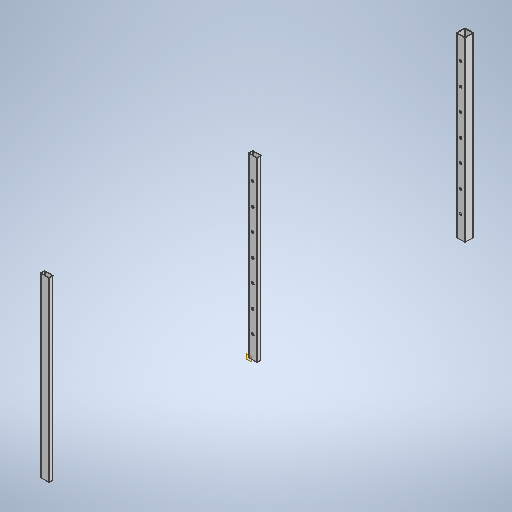
# Autodesk Inventor part: korlat1
Saved by Autodesk Inventor 2025.2 (Build 292293000, 293)
## iProperties
Created: 2025-08-30
Part Number: korlat1
Material: Generic
Document SubType Name: Modeling
Designer: MB
Density: 1 g/cm^3
Appearance: Default
Author: MB
Autodesk Inventor part; units mm, degrees
ref_plane "YZ Plane" through (0, 0, 0) normal (1, 0, 0) x (0, 1, 0)
ref_plane "XZ Plane" through (0, 0, 0) normal (0, 1, 0) x (-1, 0, 0)
ref_plane "XY Plane" through (0, 0, 0) normal (0, 0, 1) x (1, 0, 0)
sketch "Sketch1" plane through (0, 0, 0) normal (0, 1, 0) x (-1, 0, 0)
  line L0 (2, 0) -> (38, 0)
  line L1 (40, 2) -> (40, 38)
  line L2 (38, 40) -> (2, 40)
  line L3 (0, 38) -> (0, 2)
  line L4 (5, 37) -> (35, 37)
  line L5 (37, 35) -> (37, 5)
  line L6 (35, 3) -> (5, 3)
  line L7 (3, 5) -> (3, 35)
  arc A0 (5, 37) -> (3, 35) centre (5, 35) ccw
  arc A1 (37, 35) -> (35, 37) centre (35, 35) ccw
  arc A2 (3, 5) -> (5, 3) centre (5, 5) ccw
  arc A3 (35, 3) -> (37, 5) centre (35, 5) ccw
  arc A4 (38, 0) -> (40, 2) centre (38, 2) ccw
  arc A5 (0, 2) -> (2, 0) centre (2, 2) ccw
  arc A6 (2, 40) -> (0, 38) centre (2, 38) ccw
  arc A7 (40, 38) -> (38, 40) centre (38, 38) ccw
  point P0 (0, 0)
  point P1 (40, 40)
  point P2 (40, 0)
  point P3 (0, 40)
  dimension "d0" = 40
  dimension "d1" = 40
  dimension "d2" = 3
  dimension "d3" = 3
  dimension "d4" = 3
  dimension "d5" = 3
  dimension "d6" = 2
  constraints: 16 end point, 16 point on circle, 16 tangent, 8 centre point, 8 point on line, 7 equal radius, 4 parallel, 2 horizontal, 2 perpendicular
  measures "d0" distance of point (0, 40) point (40, 40)
  measures "d1" distance of point (40, 40) point (40, 0)
  measures "d2" distance between parallel lines of L0 L6
  measures "d3" distance between parallel lines of L3 L7
  measures "d4" distance between parallel lines of L1 L5
  measures "d5" distance between parallel lines of L2 L4
  measures "d6" radius of A0
extrude "Extrusion1" add sketch "Sketch1" along normal blind 800
sketch "Sketch2" plane through (-38, 0, 40) normal (0, 0, 1) x (1, 0, 0)
  line L0 (0, 0) -> (0, 800) projected
  line L1 (-2, 0) -> (-2, 800) projected
  line L2 (0, 800) -> (36, 800) projected
  point P0 (38, 0)
  point P1 (18, 700)
  point P2 (18, 800)
  point P3 (18, 600)
  point P4 (18, 500)
  point P5 (18, 400)
  point P6 (18, 300)
  point P7 (18, 200)
  point P8 (18, 100)
  dimension "d10" = 20
  dimension "d11" = 100
  dimension "d14" = 100
  constraints: 1 midpoint, 1 vertical, 6 other
  measures "d10" distance from line of L1 point (18, 700)
  measures "d11" distance of point (18, 800) point (18, 700)
  measures "d14" distance of point (18, 700) point (18, 600)
hole "Hole1" at (-20, 600, 40) at (-20, 500, 40) at (-20, 400, 40) at (-20, 300, 40) at (-20, 200, 40) at (-20, 100, 40) at (-20, 700, 40) direction (0, 0, -1) diameter 12 depth 8 tip angle 118
sketch "Sketch3" plane through (0, 0, 0) normal (0, 1, 0) x (-1, 0, 0)
  line L0 (2, 960) -> (38, 960)
  line L1 (40, 962) -> (40, 978)
  line L2 (38, 980) -> (2, 980)
  line L3 (0, 978) -> (0, 962)
  line L4 (4, 962) -> (36, 962)
  line L5 (38, 964) -> (38, 976)
  line L6 (36, 978) -> (4, 978)
  line L7 (2, 976) -> (2, 964)
  line L8 (38, 40) -> (2, 40) projected
  line L9 (0, 38) -> (0, 2) projected
  arc A0 (2, 964) -> (4, 962) centre (4, 964) ccw
  arc A1 (0, 962) -> (2, 960) centre (2, 962) ccw
  arc A2 (38, 960) -> (40, 962) centre (38, 962) ccw
  arc A3 (36, 962) -> (38, 964) centre (36, 964) ccw
  arc A4 (40, 978) -> (38, 980) centre (38, 978) ccw
  arc A5 (38, 976) -> (36, 978) centre (36, 976) ccw
  arc A6 (4, 978) -> (2, 976) centre (4, 976) ccw
  arc A7 (2, 980) -> (0, 978) centre (2, 978) ccw
  line L10 (2, 1900) -> (38, 1900)
  line L11 (40, 1902) -> (40, 1918)
  line L12 (38, 1920) -> (2, 1920)
  line L13 (0, 1918) -> (0, 1902)
  line L14 (4, 1902) -> (36, 1902)
  line L15 (38, 1904) -> (38, 1916)
  line L16 (36, 1918) -> (4, 1918)
  line L17 (2, 1916) -> (2, 1904)
  arc A8 (2, 1904) -> (4, 1902) centre (4, 1904) ccw
  arc A9 (0, 1902) -> (2, 1900) centre (2, 1902) ccw
  arc A10 (38, 1900) -> (40, 1902) centre (38, 1902) ccw
  arc A11 (36, 1902) -> (38, 1904) centre (36, 1904) ccw
  arc A12 (40, 1918) -> (38, 1920) centre (38, 1918) ccw
  arc A13 (38, 1916) -> (36, 1918) centre (36, 1916) ccw
  arc A14 (4, 1918) -> (2, 1916) centre (4, 1916) ccw
  arc A15 (2, 1920) -> (0, 1918) centre (2, 1918) ccw
  point P0 (0, 0)
  point P1 (40, 980)
  point P2 (40, 960)
  point P3 (0, 980)
  point P4 (20, 40)
  point P5 (40, 1920)
  point P6 (40, 1900)
  point P7 (0, 1920)
  point P8 (20, 980)
  dimension "d26" = 40
  dimension "d27" = 20
  dimension "d28" = 920
  dimension "d29" = 0
  dimension "d30" = 2
  dimension "d31" = 2
  dimension "d32" = 2
  dimension "d33" = 2
  dimension "d34" = 2
  dimension "d53" = 40
  dimension "d54" = 20
  dimension "d55" = 2
  dimension "d56" = 2
  dimension "d57" = 2
  dimension "d58" = 2
  dimension "d59" = 2
  dimension "d60" = 920
  constraints: 32 end point, 32 point on circle, 32 tangent, 16 centre point, 14 equal radius, 12 point on line, 8 parallel, 4 horizontal, 4 perpendicular, 2 midpoint
  measures "d26" distance of point (0, 980) point (40, 980)
  measures "d27" distance of point (40, 980) point (40, 960)
  measures "d28" distance from line of point (20, 40) L0
  measures "d29" distance between parallel lines of L9 L3
  measures "d30" distance between parallel lines of L0 L4
  measures "d31" distance between parallel lines of L1 L5
  measures "d32" distance between parallel lines of L2 L6
  measures "d33" distance between parallel lines of L3 L7
  measures "d34" radius of A0
  measures "d53" distance of point (0, 1920) point (40, 1920)
  measures "d54" distance of point (40, 1920) point (40, 1900)
  measures "d55" distance between parallel lines of L10 L14
  measures "d56" distance between parallel lines of L11 L15
  measures "d57" distance between parallel lines of L12 L16
  measures "d58" distance between parallel lines of L13 L17
  measures "d59" radius of A8
  measures "d60" distance from line of L10 point (20, 980)
ref_plane "Work Plane1" through (-38, 0, 980) normal (0, 0, 1) x (1, 0, 0)
sketch "Sketch4" plane through (-38, 0, 980) normal (0, 0, 1) x (1, 0, 0)
  line L0 (0, 800) -> (36, 800) projected
  line L1 (-2, 0) -> (-2, 800) projected
  point P0 (38, 0)
  point P1 (18, 700)
  point P2 (18, 600)
  point P3 (18, 500)
  point P4 (18, 400)
  point P5 (18, 300)
  point P6 (18, 200)
  point P7 (18, 100)
  dimension "d37" = 100
  dimension "d38" = 20
  dimension "d41" = 100
  constraints: 1 vertical, 6 other
  measures "d37" distance from line of L0 point (18, 700)
  measures "d38" distance from line of L1 point (18, 700)
  measures "d41" distance of point (18, 700) point (18, 600)
extrude "Extrusion3" add sketch "Sketch3" along normal blind 800
hole "Hole3" at (-20, 700, 980) at (-20, 600, 980) at (-20, 500, 980) at (-20, 400, 980) at (-20, 300, 980) at (-20, 200, 980) at (-20, 100, 980) direction (0, 0, -1) diameter 12 end through all
body "Solid1"
